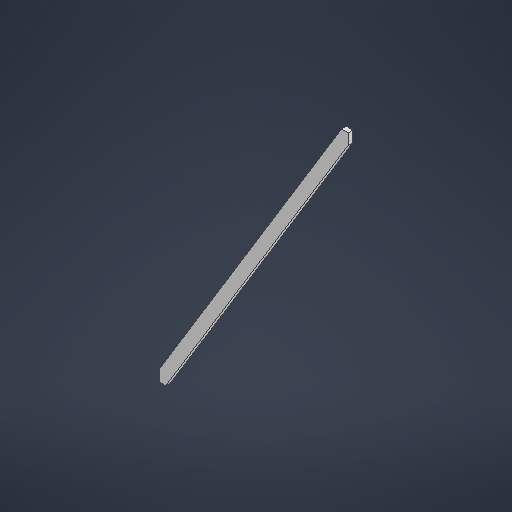
# Autodesk Inventor part: S_2x4x112.420
Saved by Autodesk Inventor 2026 (Build 300175000, 175)
## iProperties
Created: 2025-09-05
Part Number: S_2x4x112.420
Material: Generic
Document SubType Name: Modeling
Designer: trott
Density: 1 g/cm^3
Appearance: Default
Author: trott
Autodesk Inventor part; units mm, degrees
ref_plane "YZ Plane" through (0, 0, 0) normal (1, 0, 0) x (0, 1, 0)
ref_plane "XZ Plane" through (0, 0, 0) normal (0, 1, 0) x (-1, 0, 0)
ref_plane "XY Plane" through (0, 0, 0) normal (0, 0, 1) x (1, 0, 0)
sketch "Sketch1" plane through (0, 0, 0) normal (0, 0, 1) x (1, 0, 0)
  line L0 (-1177.925, -1219.2) -> (1177.925, -1219.2)
  line L1 (1177.925, -1219.2) -> (1177.925, 1219.2)
  line L2 (1177.925, 1219.2) -> (-1177.925, 1219.2)
  line L3 (-1177.925, 1219.2) -> (-1177.925, -1219.2)
  line L4 (-1177.925, -1219.2) -> (1177.925, 1219.2) construction
  line L5 (1177.925, -1219.2) -> (-1177.925, 1219.2) construction
  line L6 (-1177.925, -1219.2) -> (-307.975, -1219.2)
  line L7 (-307.975, -1219.2) -> (-307.975, 1219.2)
  line L8 (1177.925, 1219.2) -> (-307.975, -1219.2)
  line L9 (-1177.925, 1219.2) -> (-307.975, -1219.2)
  line L10 (-345.9327, -1196.0695) -> (-270.0173, -1242.3305)
  line L11 (-349.8404, -1234.1363) -> (-266.1096, -1204.2637)
  line L12 (-1219.7904, 1204.2637) -> (-1136.0596, 1234.1363)
  line L13 (1215.8827, 1196.0695) -> (1139.9673, 1242.3305)
  line L14 (1139.9673, 1242.3305) -> (-345.9327, -1196.0695)
  line L15 (-270.0173, -1242.3305) -> (1215.8827, 1196.0695)
  line L16 (-266.1096, -1204.2637) -> (-1136.0596, 1234.1363)
  line L17 (-1219.7904, 1204.2637) -> (-349.8404, -1234.1363)
  point P0 (0, 0)
  point P1 (-307.975, -1086.9184)
  point P2 (-1130.7308, 1219.2)
  point P3 (-1177.925, 1086.9184)
  point P4 (-355.1692, -1219.2)
  point P5 (-307.975, -1219.2)
  point P6 (-307.975, -1133.78)
  point P7 (1125.8722, 1219.2)
  point P8 (-255.9222, -1219.2)
  point P9 (1177.925, 1133.78)
  dimension "d0" = 2355.85
  dimension "d1" = 2438.4
  dimension "d2" = 869.95
  dimension "d3" = 88.9
  dimension "d4" = 88.9
  dimension "d6" = 88.9
  dimension "d7" = 88.9
  constraints: 36 end point, 6 midpoint, 6 perpendicular, 2 parallel, 2 point on line, 1 horizontal
  measures "d0" distance of L2.end L1.end
  measures "d1" distance of L0.end L1.end
  measures "d2" distance of L0.start L6.end
  measures "d3" distance of L10.start L10.end
  measures "d4" distance of L11.start L11.end
  measures "d6" distance of L12.start L12.end
  measures "d7" distance of L13.start L13.end
extrude "Extrusion1" add sketch "Sketch1" along normal blind 38.1 contours L11 L16 L8 L1 L15 L0 | L7 L14 L16 L8 | L8 L16 L11 | L16 L14 L2 L8
body "Solid1"
